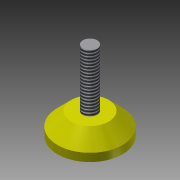
# Autodesk Inventor part: 23015T82
Saved by Autodesk Inventor 2013 SP2 (Build 170200200, 200)
## iProperties
Created: 2013-05-31
Part Number: 23015T82
Material: Generic
Document SubType Name: Modeling
Designer: Edward
Density: 1 g/cm^3
Description: leveling feet, 1/4" x 20 Threaded Stud
Vendor: mcmaster
Catalog Web Link: http://www.mcmaster.com/#catalog/119/1360/=mzp82c
Mass: 5.52311 g
Surface Area: 22.8201 cm^2
Volume: 5.52311 cm^3
Stock Number: 23015T82
Author: Edward
Autodesk Inventor part; units mm, degrees
ref_plane "YZ Plane" through (0, 0, 0) normal (1, 0, 0) x (0, 1, 0)
ref_plane "XZ Plane" through (0, 0, 0) normal (0, 1, 0) x (-1, 0, 0)
ref_plane "XY Plane" through (0, 0, 0) normal (0, 0, 1) x (1, 0, 0)
sketch "Sketch1" plane through (0, 0, 0) normal (0, 0, 1) x (1, 0, 0)
  circle A0 centre (0, 0) radius 14.2875
  dimension "d0" = 28.575
  constraints: 1 centre point, 1 coincident
  measures "d0" diameter of A0
extrude "Extrusion1" add sketch "Sketch1" along normal blind 9.525
sketch "Sketch2" plane through (0, 0, 9.525) normal (0, 0, 1) x (1, 0, 0)
  circle A0 centre (0, 0) radius 14.2875 projected
  circle A1 centre (0, 0) radius 3.175
  dimension "d4" = 6.35
  constraints: 1 centre point, 1 coincident
  measures "d4" diameter of A1
extrude "Extrusion2" add sketch "Sketch2" along normal blind 25.4 contours A1
chamfer "Chamfer1" distance 6 angle 45 1 edges at (-14.2875, 0, 9.525)
thread "Thread1" size "1/4-20 UNC" class "2A" standard "ANSI Unified Screw Threads" full length
body "Solid1"
